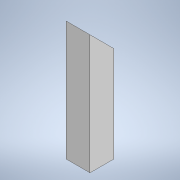
# Autodesk Inventor part: Viewing Mirror Holder
Saved by Autodesk Inventor 2022 (Build 260153000, 153)
## iProperties
Created: 2023-09-18
Part Number: Viewing Mirror Holder
Material: Generic
Document SubType Name: Modeling
Designer: fouad
Density: 1 g/cm^3
Appearance: Default
Author: fouad
Autodesk Inventor part; units mm, degrees
ref_plane "YZ Plane" through (0, 0, 0) normal (1, 0, 0) x (0, 1, 0)
ref_plane "XZ Plane" through (0, 0, 0) normal (0, 1, 0) x (-1, 0, 0)
ref_plane "XY Plane" through (0, 0, 0) normal (0, 0, 1) x (1, 0, 0)
sketch "Sketch2" plane through (0, 0, 0) normal (0, 1, 0) x (-1, 0, 0)
  line L0 (2.5667, 3.1167) -> (0.5667, 3.1167)
  line L1 (0.5667, 3.1167) -> (0.5667, 1.1167)
  line L2 (0.5667, 1.1167) -> (2.5667, 1.1167)
  line L3 (2.5667, 1.1167) -> (2.5667, 3.1167)
  point P0 (0, 0)
  dimension "d5" = 2
  dimension "d6" = 2
  constraints: 8 end point, 2 parallel, 1 horizontal, 1 perpendicular
  measures "d5" distance of L2.end L1.end
  measures "d6" distance of L1.end L0.end
extrude "Extrusion1" add sketch "Sketch2" along normal blind 10
sketch "Sketch3" plane through (-0.5667, 0, 3.1167) normal (1, 0, 0) x (0, 0, -1)
  line L0 (0, 10) -> (2, 10) projected
  line L1 (0, 10) -> (2, 8)
  line L2 (2, 0) -> (2, 10) projected
  line L3 (0, 10) -> (2.8284, 10) construction
  point P0 (3.1167, 0)
  dimension "d9" = 45
  constraints: 4 end point, 1 equal length, 1 horizontal, 1 point on line
  measures "d9" angle of L1 L3
extrude "Extrusion2" cut sketch "Sketch3" against normal through all
body "Solid1"
